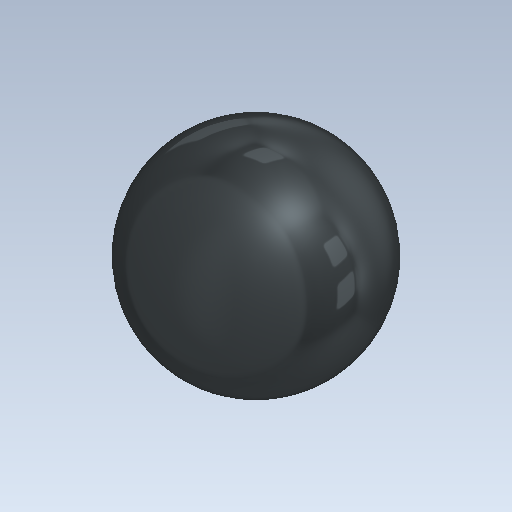
# Autodesk Inventor part: 040205DR-19-H6_ball
Saved by Autodesk Inventor 2021.2 (Build 252289000, 289)
## iProperties
Part Number: 040205DR-19-H6_ball
Material: 鉄、鋳鉄
Catalog Web Link: www.cadenas.de
Description: DR-H ball-D-Series bearings
Vendor: TOKBEARING
Document SubType Name: Modeling
Designer: partserver
Manufacturer: TOKBEARING
Mass: 8100 g
Surface Area: 0.294166 cm^2
Volume: 0.0150025 cm^3
Density: 7.15 g/cm^3
Appearance: 鉄 灰色
Category: PARTsolutions
Company: TOKBEARING
PSOL_IDENT_0: {$CADENAS_DATA\23d-libs\tok_bearing\d_series_bearings\dr_h\dr_h_ball.prj},183 {VTYP=3D},{NB=040205DR
PSOL_IDENT_1: -19-H6_ball},{LINA=040205DR-19-H6_ball},{NN=DR-H ball},{DATE=16.12.2020 00:38:04},{GEOMDATE=19.02.20
PSOL_IDENT_2: 13 00:00:00},{VERSION=},{LINEID=1520},{WBVAR=},{WBNUMERIC=}  {NB=040205DR-19-H6_ball},{LINA=040205DR
PSOL_IDENT_3: -19-H6_ball},{KT=DUMMY},{IDNR=},{CODE=040205},{PN=DR-19-H6},{D=19},{SD=6.0},{W=6.0},{W1=-},{W1X=0.00
PSOL_IDENT_4: 0},{W2=-},{W2X=0.000},{LOAD=49 (5)},{TYPE=10},{QTY=2.500},{GW=8.1},{BD=3.06},{OP=35.2622},{N=5},{R=5
PSOL_IDENT_5: .615},{GP=3.12}
NB: 040205DR-19-H6_ball
NN: DR-H ball
NT: D-Series bearings
NBSYN: $CODE.$PN._ball
LINA: 040205DR-19-H6_ball
CATALOG: TOK, Inc
CODE: 040205
PN: DR-19-H6
D: 19
SD: 6
W: 6
W1: -
W2: -
LOAD: 49 (5)
TYPE: 10
QTY: 2.500
GW: 8.1
SUPPLIER: TOKBEARING
ARTICLENO: 040205DR-19-H6_ball
BOMINFO: 040205DR-19-H6_ball
CREATOR: CADENAS GmbH
Title: 040205DR-19-H6_ball
Author: Cadenas PARTsolutions
Comments: D-Series bearings
Autodesk Inventor part; units mm, degrees
sketch "Sketch_1" plane through (0, 0, 0) normal (0, 0, 1) x (1, 0, 0)
  line L0 (1.53, 0) -> (-1.53, 0)
  arc A0 (1.53, 0) -> (-1.53, 0) centre (0, 0) ccw
  line L1 (1.53, 0) -> (-1.53, 0)
  constraints: 4 end point, 2 point on circle, 1 centre point
revolve "Revolution1" add sketch "Sketch_1" angle 360 about axis through (1.53, 0, 0) along (1, 0, 0)
ref_plane "Ball_OR_XY" through (0, 0, 0) normal (1, 0, 0) x (0, 0, -1)
ref_plane "Ball_OR_YZ" through (0, 0, 0) normal (0, 0, -1) x (0, 1, 0)
ref_plane "Ball_OR_ZX" through (0, 0, 0) normal (0, 1, 0) x (1, 0, 0)
body "Solid1"
